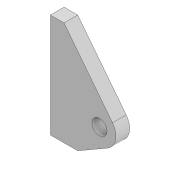
# Autodesk Inventor part: Catch plate
Saved by Autodesk Inventor 2020.1 (Build 241239000, 239)
## iProperties
Created: 2019-10-07
Part Number: Catch plate
Material: Generic
Document SubType Name: Modeling
Designer: thom_tremblay
Density: 1 g/cm^3
Appearance: Default
Author: thom_tremblay
Autodesk Inventor part; units mm, degrees
ref_plane "YZ Plane" through (0, 0, 0) normal (1, 0, 0) x (0, 1, 0)
ref_plane "XZ Plane" through (0, 0, 0) normal (0, 1, 0) x (-1, 0, 0)
ref_plane "Work Plane1" through (0, 0, 0) normal (0, 0, 1) x (1, 0, 0)
sketch "Sketch1" plane through (0, 0, 0) normal (0, 0, 1) x (1, 0, 0)
  line L0 (0, 0) -> (0, -96.52)
  line L1 (0, -96.52) -> (25.4, -96.52)
  line L2 (25.4, -96.52) -> (53.34, -80.3888)
  arc A0 (53.34, -80.3888) -> (57.7429, -57.8254) centre (45.72, -67.1906) ccw
  line L3 (57.7429, -57.8254) -> (12.7, 0)
  line L4 (12.7, 0) -> (0, 0)
  dimension "d0" = 96.52
  dimension "d1" = 25.4
  dimension "d2" = 60.96
  dimension "d3" = 15.24
  dimension "d4" = 12.7
  dimension "d5" = 30
  constraints: 10 end point, 2 point on circle, 2 tangent, 1 centre point, 1 parallel, 1 perpendicular, 1 vertical
  measures "d0" distance of L0.start L0.end
  measures "d1" distance of L0.end L1.end
  measures "d3" radius of A0
  measures "d4" distance of L3.end L0.start
  measures "d5" angle of L1 L2
extrude "Extrusion1" add sketch "Sketch1" along normal mid plane 12.7
sketch "Sketch2" plane through (0, 0, 6.35) normal (0, 0, 1) x (1, 0, 0)
  arc A0 (53.34, -80.3888) -> (57.7429, -57.8254) centre (45.72, -67.1906) ccw projected
  point P0 (0, 0)
  constraints: 1 coincident
hole "Hole1" at (45.72, -67.1906, 6.35) direction (0, 0, -1) diameter 13.8938 end through all clearance for "Flat Head Machine Screw (82)" size "1/2" standard "Ansi Unified Screw Threads"
body "Solid1"
